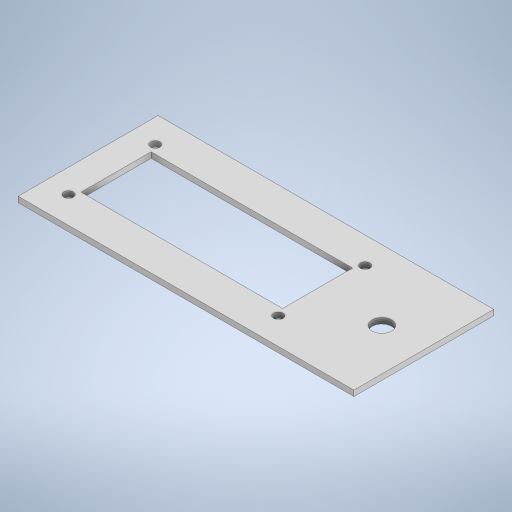
# Autodesk Inventor part: Bedienfeld
Saved by Autodesk Inventor 2023.1 (Build 271208000, 208)
## iProperties
Created: 2023-04-27
Part Number: Bedienfeld
Material: Generisch
Document SubType Name: Sheet Metal
Designer: marco
Density: 1 g/cm^3
Sheet Metal Rule: Standard_mm
Appearance: Vorgabe
Author: marco
Autodesk Inventor part; units mm, degrees
ref_plane "YZ Plane" through (0, 0, 0) normal (1, 0, 0) x (0, 1, 0)
ref_plane "XZ Plane" through (0, 0, 0) normal (0, 1, 0) x (-1, 0, 0)
ref_plane "XY Plane" through (0, 0, 0) normal (0, 0, 1) x (1, 0, 0)
sketch "Skizze1" plane through (0, 0, 0) normal (0, 1, 0) x (-1, 0, 0)
  line L0 (0, 0) -> (120, 0)
  line L1 (120, 0) -> (120, -50)
  line L2 (120, -50) -> (0, -50)
  line L3 (0, -50) -> (0, 0)
  line L4 (110, -37.5) -> (38, -37.5)
  line L5 (38, -37.5) -> (38, -12.5)
  line L6 (38, -12.5) -> (110, -12.5)
  line L7 (110, -12.5) -> (110, -37.5)
  line L8 (114, -43) -> (34, -43)
  line L9 (34, -43) -> (34, -7)
  line L10 (34, -7) -> (114, -7)
  line L11 (114, -7) -> (114, -43)
  circle A0 centre (111.5, -40.5) radius 1.7
  circle A1 centre (36.5, -40.5) radius 1.7
  circle A2 centre (111.5, -9.5) radius 1.7
  circle A3 centre (36.5, -9.5) radius 1.7
  circle A4 centre (15, -25) radius 3.5
  dimension "d0" = 120
  dimension "d1" = 50
  dimension "d2" = 72
  dimension "d3" = 25
  dimension "d4" = 80
  dimension "d5" = 36
  dimension "d6" = 5.5
  dimension "d7" = 5.5
  dimension "d8" = 4
  dimension "d9" = 4
  dimension "d10" = 3.4
  dimension "d11" = 3.4
  dimension "d12" = 75
  dimension "d13" = 2.5
  dimension "d14" = 2.5
  dimension "d15" = 3.4
  dimension "d16" = 3.4
  dimension "d17" = 2.5
  dimension "d18" = 2.5
  dimension "d19" = 31
  dimension "d20" = 2.5
  dimension "d21" = 2.5
  dimension "d22" = 2.5
  dimension "d23" = 7
  dimension "d24" = 7
  dimension "d25" = 15
  dimension "d26" = 6
  constraints: 24 end point, 6 parallel, 5 centre point, 3 horizontal, 3 perpendicular
  measures "d0" distance of L1.end L2.end
  measures "d1" distance of L0.end L1.end
  measures "d2" distance of L5.end L6.end
  measures "d3" distance of L4.end L5.end
  measures "d4" distance of L9.end L10.end
  measures "d5" distance of L8.end L9.end
  measures "d6" distance between parallel lines of L8 L4
  measures "d7" distance between parallel lines of L6 L10
  measures "d8" distance between parallel lines of L9 L5
  measures "d9" distance between parallel lines of L11 L7
  measures "d10" diameter of A0
  measures "d11" diameter of A1
  measures "d12" distance of A0.centre A1.centre
  measures "d13" distance from line of L11 A0.centre
  measures "d14" distance from line of L9 A1.centre
  measures "d15" diameter of A2
  measures "d16" diameter of A3
  measures "d17" distance from line of L8 A0.centre
  measures "d18" distance from line of L8 A1.centre
  measures "d19" distance of A2.centre A0.centre
  measures "d20" distance from line of L10 A3.centre
  measures "d21" distance from line of L11 A2.centre
  measures "d22" distance from line of L9 A3.centre
  measures "d23" distance between parallel lines of L2 L8
  measures "d24" diameter of A4
  measures "d25" distance from line of L3 A4.centre
  measures "d26" distance between parallel lines of L1 L11
extrude "Extrusion1" add sketch "Skizze1" along normal blind 2 contours L0 L1 L2 L3 | L8 L9 L10 L11
equation "\"d10\" = d15"
equation "\"d11\" = d15"
equation "\"d16\" = d15"
equation "\"Biegeradius\" = Stärke"
equation "\"BreiteBiegungsfreistellung\" = Stärke"
equation "\"TiefeBiegungsfreistellung\" = 0.5 * Stärke"
equation "\"GrößeEckenfreistellung\" = 4 * Stärke"
equation "\"MinimalRest\" = 2 * Stärke"
equation "\"Übergangsradius\" = Biegeradius"
equation "\"JacobiRadiusGröße\" = Biegeradius"
equation "\"Abstandsgröße\" = Stärke"
equation "\"Stärke\" = 0.5"
